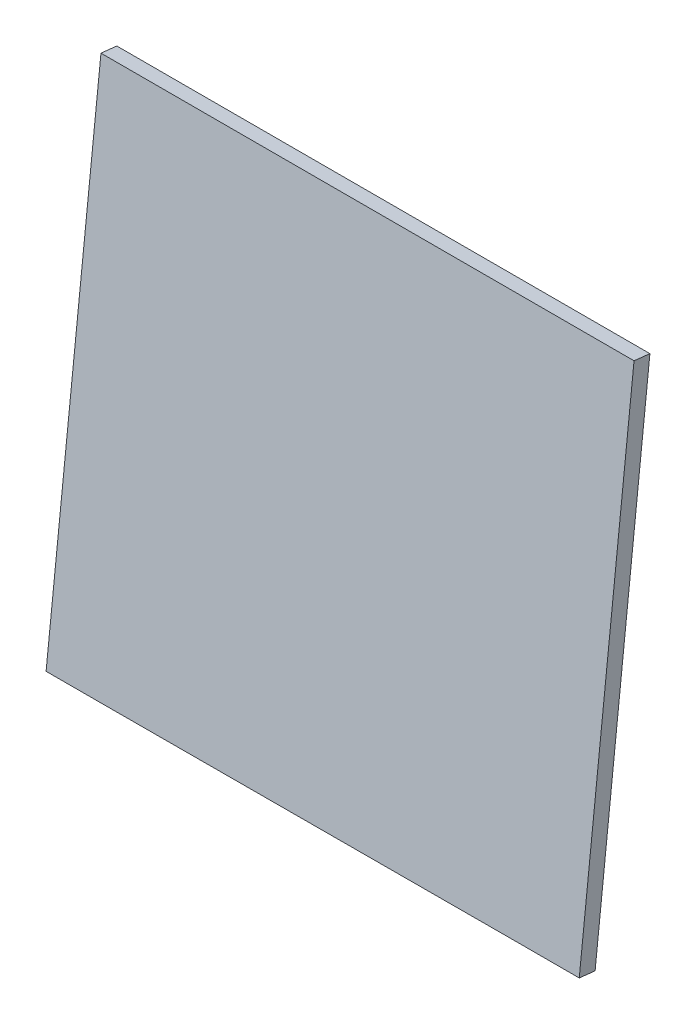
# Autodesk Inventor part: Top Plate
Saved by Autodesk Inventor 2023.2 (Build 272271000, 271)
## iProperties
Created: 2023-01-31
Part Number: Top Plate
Material: Aluminum 6061
Document SubType Name: Modeling
Designer: dmargari
Density: 2.7 g/cm^3
Appearance: Aluminum - Flat
Mass: 95.25 g
Surface Area: 408.7 cm^2
Volume: 95.25 cm^3
Author: dmargari
Autodesk Inventor part; units mm, degrees
ref_plane "YZ Plane" through (0, 0, 0) normal (1, 0, 0) x (0, 1, 0)
ref_plane "XZ Plane" through (0, 0, 0) normal (0, 1, 0) x (-1, 0, 0)
ref_plane "XY Plane" through (0, 0, 0) normal (0, 0, 1) x (1, 0, 0)
ref_plane "Work Plane1" through (1137.1683, -307183.6325, 62520.3196) normal (-0.0000273, 0.1077029, 0.9941831) x (1, 0.0002593, -0.0000006)
sketch "Sketch1" plane through (1137.1683, -307183.6325, 62520.3196) normal (-0.0000273, 0.1077029, 0.9941831) x (1, 0.0002593, -0.0000006)
  line L0 (0.9152, -7.9083) -> (121.915, -7.6807) projected
  line L1 (0.9152, -7.9083) -> (-2.0848, -7.9139) projected
  line L2 (124.915, -7.675) -> (121.915, -7.6807) projected
  line L3 (124.915, -7.7516) -> (-2.0848, -7.7516)
  line L4 (124.915, -7.675) -> (144.915, -7.675)
  line L5 (144.915, -7.675) -> (144.915, 152.0861)
  line L6 (-2.0848, -7.9139) -> (-22.0848, -7.9139)
  line L7 (-2.0848, -7.9139) -> (17.9152, -7.9139) construction
  line L8 (-22.0848, -7.9139) -> (-22.0848, 152.0861)
  line L9 (-22.0848, 152.0861) -> (144.915, 152.0861)
  point P0 (-1057.4924, 312130.6861)
  dimension "d5" = 20
  dimension "d8" = 20
  dimension "d9" = 180
  dimension "d10" = 160
  dimension "d11" = 90
  dimension "d12" = 166.9998
  constraints: 14 end point, 4 horizontal, 3 perpendicular, 1 collinear
  measures "d5" distance of L2.start L4.end
  measures "d8" distance of L1.end L6.end
  measures "d9" angle of L6 L7
  measures "d10" distance of L6.end L8.end
  measures "d11" angle of L6 L8
  measures "d12" distance of L8.end L5.end
extrude "Extrusion1" add sketch "Sketch1" along normal blind 5
body "Solid1"
